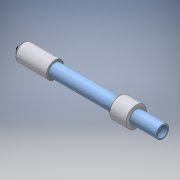
# Autodesk Inventor part: PH Monitor
Saved by Autodesk Inventor 2016 (Build 200138000, 138)
## iProperties
Created: 2016-02-27
Part Number: PH Monitor
Material: Generic
Document SubType Name: Modeling
Designer: Kenneth Daniel
Density: 1 g/cm^3
Appearance: Default
Mass: 26.7988 g
Surface Area: 80.8969 cm^2
Volume: 26.7988 cm^3
Author: Kenneth Daniel
Autodesk Inventor part; units mm, degrees
ref_plane "YZ Plane" through (0, 0, 0) normal (1, 0, 0) x (0, 1, 0)
ref_plane "XZ Plane" through (0, 0, 0) normal (0, 1, 0) x (-1, 0, 0)
ref_plane "XY Plane" through (0, 0, 0) normal (0, 0, 1) x (1, 0, 0)
sketch "Sketch1" plane through (0, 0, 0) normal (0, 0, 1) x (1, 0, 0)
  line L0 (-31, 6.1) -> (0, 6.1)
  line L1 (0, 6.1) -> (31, 6.1)
  line L2 (0, 10.5424) -> (0, 0) construction
  line L3 (31, 9.75) -> (31, 6.1)
  line L4 (77, 9.75) -> (77, 0)
  line L5 (46.4247, 9.75) -> (46.4247, 4.1503)
  line L6 (46.4247, 4.1503) -> (48.4247, 4.1503)
  line L7 (48.4247, 4.1503) -> (48.4247, 9.75)
  line L8 (31, 9.75) -> (46.4247, 9.75) construction
  line L9 (31, 9.75) -> (46.4247, 9.75)
  line L10 (62.7124, 9.75) -> (62.7124, 9.1289)
  line L11 (62.7124, 9.1289) -> (62.9117, 9.1289)
  line L12 (62.9117, 9.1289) -> (62.9117, 9.75)
  line L13 (48.4247, 9.75) -> (62.7124, 9.75) construction
  line L14 (62.9117, 9.75) -> (77, 9.75) construction
  line L15 (48.4247, 9.75) -> (62.7124, 9.75)
  line L16 (62.9117, 9.75) -> (77, 9.75)
  line L17 (-31, 8.1) -> (-60.2, 8.1)
  line L18 (-60.2, 8.1) -> (-60.2, 0)
  line L19 (-31, 8.1) -> (-31, 6.1)
  line L20 (-60.2, 4.875) -> (-63.45, 4.875)
  line L21 (-66.7, 0) -> (-60.2, 0)
  line L22 (-63.45, 4.875) -> (-63.45, 2.7274)
  line L23 (-63.45, 2.7274) -> (-65.075, 2.7274)
  line L24 (-65.075, 2.7274) -> (-65.075, 1.425)
  line L25 (-65.075, 1.425) -> (-66.7, 1.425)
  line L26 (-66.7, 1.425) -> (-66.7, 0)
  line L27 (-60.2, 0) -> (77, 0)
  line L28 (-95.44, 0) -> (105.74, 0) projected
  dimension "d1" = 31
  dimension "d2" = 31
  dimension "d3" = 6.1
  dimension "d4" = 46
  dimension "d6" = 2
  dimension "d7" = 29.2
  dimension "d8" = 8.1
  dimension "d10" = 1.425
  dimension "d11" = 6.5
  constraints: 56 end point, 15 perpendicular, 8 horizontal, 8 vertical, 2 point on line, 1 other
  measures "d1" distance of L0.end L0.start
  measures "d2" distance of L1.end L0.end
  measures "d3" distance of L2.end L0.end
  measures "d4" distance of L3.start L4.start
  measures "d6" distance of L5.end L6.end
  measures "d7" distance of L17.start L17.end
  measures "d8" distance from line of L2.end L17
  measures "d10" distance from line of L21 L24.end
  measures "d11" distance of L21.start L18.end
revolve "Revolution1" add sketch "Sketch1" angle 360 about axis through (-10, 0, 0) along (1, 0, 0)
sketch "Sketch2" plane through (77, 0, 0) normal (1, 0, 0) x (0, 0, -1)
  circle A0 centre (0, 0) radius 9.75 projected
extrude "Extrusion1" cut sketch "Sketch2" against normal up to surface (30.5753 mm away)
sketch "Sketch3" plane through (46.4247, 0, 0) normal (1, 0, 0) x (0, 0, -1)
  circle A0 centre (0, 0) radius 6.1
  dimension "d15" = 12.2
  constraints: 1 centre point, 1 coincident
  measures "d15" diameter of A0
extrude "Extrusion2" add sketch "Sketch3" along normal blind 25
sketch "Sketch4" plane through (71.4247, 0, 0) normal (1, 0, 0) x (0, 0, -1)
  circle A0 centre (0, 0) radius 4.875
  circle A1 centre (0, 0) radius 6.1 projected
  line L0 (0, 0) -> (0, 10.6003)
  line L1 (0, 0) -> (6.8931, 6.8955)
  circle A2 centre (0, 0) radius 9.75 projected
  circle A3 centre (0, 0) radius 8.1
  circle A4 centre (0, 0) radius 9.75
  constraints: 4 end point, 3 centre point, 3 coincident, 1 vertical, 2 other
extrude "Extrusion3" cut sketch "Sketch4" against normal blind 5 contours A0 L0 L1 | L1 L0 A0
body "Solid1"
